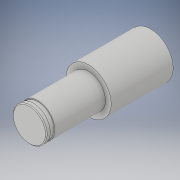
# Autodesk Inventor part: Component 3 (Planet Gear Axis)
Saved by Autodesk Inventor 2018 (Build 220112000, 112)
## iProperties
Created: 2023-03-14
Part Number: Component 3 (Planet Gear Axis)
Material: Generic
Document SubType Name: Modeling
Designer: Habib Mohamed
Density: 1 g/cm^3
Appearance: Default
Author: Habib Mohamed
Autodesk Inventor part; units mm, degrees
ref_plane "YZ Plane" through (0, 0, 0) normal (1, 0, 0) x (0, 1, 0)
ref_plane "XZ Plane" through (0, 0, 0) normal (0, 1, 0) x (-1, 0, 0)
ref_plane "XY Plane" through (0, 0, 0) normal (0, 0, 1) x (1, 0, 0)
sketch "Sketch1" plane through (0, 0, 0) normal (1, 0, 0) x (0, 1, 0)
  line L0 (0, 0) -> (0, -21.5)
  line L1 (0, -21.5) -> (4, -21.5)
  line L2 (4, -21.5) -> (4, -10.5)
  line L3 (4, -10.5) -> (3, -10.5)
  line L4 (3, -10.5) -> (3, -1.5)
  line L5 (3, -1.5) -> (2.85, -1.5)
  line L6 (2.85, -1.5) -> (2.85, -0.7)
  line L7 (2.85, -0.7) -> (3, -0.7)
  line L8 (3, -0.7) -> (3, -0.15)
  line L9 (3, -0.15) -> (2.85, 0)
  line L10 (2.85, 0) -> (0, 0)
  dimension "d0" = 21.5
  dimension "d1" = 0.15
  dimension "d2" = 0.15
  dimension "d3" = 0.7
  dimension "d4" = 0.15
  dimension "d5" = 0.8
  dimension "d6" = 11
  dimension "d7" = 9
  dimension "d8" = 4
  dimension "d9" = 3
  constraints: 22 end point, 7 perpendicular, 2 point on line, 1 parallel, 1 vertical
  measures "d0" distance of L0.start L0.end
  measures "d1" horizontal distance of L8.end L9.end
  measures "d2" horizontal distance of L8.end L9.end
  measures "d3" distance between parallel lines of L7 L10
  measures "d4" distance between parallel lines of L6 L8
  measures "d5" distance of L5.end L6.end
  measures "d6" distance of L1.end L2.end
  measures "d7" distance of L3.end L4.end
  measures "d8" distance between parallel lines of L2 L0
  measures "d9" distance between parallel lines of L0 L4
revolve "Revolution1" add sketch "Sketch1" angle 360 about axis through (0, 0, 0) along (0, 0, -1)
body "Solid1"
